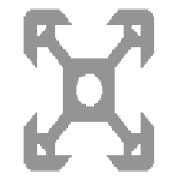
# Autodesk Inventor part: V-slot 20 mm x 20 mm
Saved by Autodesk Inventor 2019 (Build 230136000, 136)
## iProperties
Created: 2018-12-31
Part Number: V-slot 20 mm x 20 mm
Material: Aluminum 6061
Description: V Slot Extrusion
Document SubType Name: Modeling
Designer: Ax
Manufacturer: Openbuilds
Standards Organization: ISO
Language: en-US
Size Designation: 470 mm 2020 V-Slot
Categories: <MemberInstance><Categories><Category DisplayName="Structural Shapes" InternalName="089c4875-fa83-4c05-b084-43b9cc11f5ed" Mnemonic="GRDR"><CategoryParameter DisplayName="Mass per Length Unit" InternalName="0bb95a10-148f-4027-a459-38d7b056702a" Mnemonic="shpmass"/><CategoryParameter DisplayName="Section Area" InternalName="1ff91680-64b0-4202-b9a3-7fd3f94bba3b" Mnemonic="secarea"/><CategoryParameter DisplayName="Radius of Gyration (x)" InternalName="25778675-03e9-40c1-b6a8-4a9ed693320d" Mnemonic="gyrradx"/><CategoryParameter DisplayName="Torsional Rigidity Modulus" InternalName="26c1ec35-5026-4c63-ad0a-751cf684a536" Mnemonic="torrigmod"/><CategoryParameter DisplayName="Distance of the Center of Gravity X-X" InternalName="26c9bdb8-9c79-4b4f-a92e-8e197583c9c4" Mnemonic="grcendistX"/><CategoryParameter DisplayName="Legacy Member ID" InternalName="340afe4f-75d7-48d3-ab7d-943f3c3da468" Mnemonic="LegacyMemberID"/><CategoryParameter DisplayName="Base Length" InternalName="42e34263-8f20-4d0e-ad48-bf1385b87c24" Mnemonic="shplen"/><CategoryParameter DisplayName="Moment of Inertia (y)" InternalName="4b9f58ea-bced-460e-81ea-3d29ca5a49e3" Mnemonic="inermomy"/><CategoryParameter DisplayName="Moment of Inertia (x)" InternalName="4cd780bc-73d7-43ac-917a-579e5cbd684d" Mnemonic="inermomx"/><CategoryParameter DisplayName="Custom Base Point" InternalName="4f1d1b73-316d-484b-a3df-9cbabb16eb77" Mnemonic="shpBasePoint"/><CategoryParameter DisplayName="Shape Height" InternalName="50274e7d-5ac0-4796-92cb-c59e54983c67" Mnemonic="shpheig"/><CategoryParameter DisplayName="Section Module (y)" InternalName="59eaa5e9-d227-48dc-b6c1-6920f96e0f95" Mnemonic="secmody"/><CategoryParameter DisplayName="Section Designation" InternalName="5a64d034-428d-49c8-ba32-7619764de20f" Mnemonic="shpdes"/><CategoryParameter DisplayName="Section Module (x)" InternalName="72cfad18-cf51-4ed4-aaa7-c6b224f8419f" Mnemonic="secmodx"/><CategoryParameter DisplayName="Torsional Section Modulus" InternalName="7c55a8dc-8844-49f9-a867-cc677b30ec9a" Mnemonic="torsecmod"/><CategoryParameter DisplayName="Shape Width" InternalName="7c717d54-a18f-4666-b4d4-573cce22c62c" Mnemonic="shpwdth"/><CategoryParameter DisplayName="Second Shape Thickness" InternalName="9251a8e1-85fd-4e47-af99-afdb762317d9" Mnemonic="shpthick2"/><CategoryParameter DisplayName="FG Authored" InternalName="9c666724-f362-4ea7-ac62-f6a007de5c69" Mnemonic="shpFGAuto"/><CategoryParameter DisplayName="Distance of the Center of Gravity Y-Y" InternalName="bcc4fb17-7af4-436a-8f8c-d0aa3b0248c5" Mnemonic="grcendistY"/><CategoryParameter DisplayName="Radius of Gyration (y)" InternalName="bfa18ebe-1636-4dbe-8d42-b263e0b73184" Mnemonic="gyrrady"/><CategoryParameter DisplayName="Shape Thickness" InternalName="d109cf76-8eb4-42fc-9800-4409734adc67" Mnemonic="shpthick"/><CategoryParameter DisplayName="Coefficient of Shear Displacement" InternalName="de4c90c6-aaa8-468f-a335-6737b311b5d3" Mnemonic="shdispc"/><Category DisplayName="Square/Rectangular Tubes" InternalName="afc8e2d8-05d6-4609-8807-f98a9b7d2ed0" Mnemonic="SQRSHP"><CategoryParameter DisplayName="Section Area" InternalName="2f7f79dd-983c-4263-802a-5b6a1495fdc5" Mnemonic="secarea"/><CategoryParameter DisplayName="Section Module (x)" InternalName="50d965a6-04bf-46b9-8ace-861858d348e6" Mnemonic="secmodx"/><CategoryParameter DisplayName="Section Module (y)" InternalName="5106aeac-54a2-4159-a9af-8933dd39dba2" Mnemonic="secmody"/><CategoryParameter DisplayName="Shape Thickness" InternalName="52712fc5-f4ee-4eda-b3f2-6fce82c26419" Mnemonic="shpthick"/><CategoryParameter DisplayName="Moment of Inertia (y)" InternalName="55ec8510-8276-4c45-8f10-594e0fee7eb3" Mnemonic="inermomy"/><CategoryParameter DisplayName="Radius of Gyration (x)" InternalName="56c89926-a299-4389-a862-ac94c9691272" Mnemonic="gyrradx"/><CategoryParameter DisplayName="Radius" InternalName="5d8d062c-e28e-41c1-98da-8e5fee36da1a" Mnemonic="shprad"/><CategoryParameter DisplayName="Moment of Inertia (x)" InternalName="8c4637b6-6b69-4878-9d5d-26a32185d655" Mnemonic="inermomx"/><CategoryParameter DisplayName="Shape Width" InternalName="8c8a1782-5e80-4d77-858b-304b1c0ad1fd" Mnemonic="shpwdth"/><CategoryParameter DisplayName="Radius of Gyration (y)" InternalName="fa48a7f5-f030-40f9-a60b-de8a845b7104" Mnemonic="gyrrady"/></Category></Category><Category DisplayName="DataType" InternalName="23b78d0f-2648-40c6-8793-ca6db495c9e8" Mnemonic="DATATYPE"><CategoryParameter DisplayName="DisplayName" InternalName="05415f3d-3907-474b-a020-eb9d644f4cf3" Mnemonic="DISPLAYNAME"/><CategoryParameter DisplayName="Standard" InternalName="0c0a119c-1e12-4c84-803f-101930972f5e" Mnemonic="STANDARD"/><CategoryParameter DisplayName="Description" InternalName="13903e3d-64b1-4950-80da-f627842ea37f" Mnemonic="DESCRIPTION"/><CategoryParameter DisplayName="Designation" InternalName="2675968c-4ce5-49e0-a4f5-552d29089031" Mnemonic="DESIGNATION"/><CategoryParameter DisplayName="Default Row" InternalName="2af9ec52-faaa-4026-b378-f9fa4afca842" Mnemonic="DEFAULTROW"/><CategoryParameter DisplayName="Folder Name" InternalName="3f06958e-8713-4116-9be7-ed6184ecc97b" Mnemonic="FOLDERNAME"/><CategoryParameter DisplayName="Revision Guid" InternalName="45a75005-10b1-4dfc-8d6d-dfe629f0b93c" Mnemonic="REVISIONGUID"/><CategoryParameter DisplayName="FileName" InternalName="8b46a4cc-9585-4fed-90c3-899f57e09a73" Mnemonic="FILENAME"/><CategoryParameter DisplayName="StdsOrg" InternalName="8f5914e1-4693-403f-8ab5-d37768198c9d" Mnemonic="STDSORG"/><CategoryParameter DisplayName="Family Version" InternalName="914462f6-6e19-4b14-ba84-155b9680b1d0" Mnemonic="FAMILYREVISION"/><CategoryParameter DisplayName="Standard Revision" InternalName="91d5a463-65c2-4fde-b823-3b7fea5e8e17" Mnemonic="STANDARDREVISION"/><CategoryParameter DisplayName="Member Revision" InternalName="a65d44b9-392f-4f4f-857b-e4b3d54996fe" Mnemonic="MEMBERREVISION"/><CategoryParameter DisplayName="ClipFormat" InternalName="bc51e27b-3422-4e78-93ef-cec197ddf230" Mnemonic="CLIPFORMAT"/><CategoryParameter DisplayName="Manufacturer" InternalName="cd6c7a72-a28a-4e50-99a9-2c7f4e13e5ad" Mnemonic="MANUFACTURER"/><CategoryParameter DisplayName="InternalName" InternalName="cf1d0246-76d9-4b4a-8305-fa0409afb5c1" Mnemonic="INTERNALNAME"/><CategoryParameter DisplayName="IsMetric" InternalName="e2385c5b-1ea4-4823-96a8-8de651266ec3" Mnemonic="ISMETRIC"/><Category DisplayName="Part" InternalName="c0e0b642-3bcb-4cc8-9e80-f96d35c4afa4" Mnemonic="PART"><CategoryParameter DisplayName="Part Number" InternalName="016b6077-bfbe-49bd-92c9-d8d59c39c941" Mnemonic="PARTNUMBER"/><CategoryParameter DisplayName="Stock Number" InternalName="4dba7c1c-e26c-444e-836c-b08b433409a8" Mnemonic="STOCKNUMBER"/><CategoryParameter DisplayName="Material Key" InternalName="5c9a8adb-dd2b-4535-b97f-0a94a95fe41f" Mnemonic="MATERIALKEY"/><CategoryParameter DisplayName="Material" InternalName="818a152a-d3c3-49ca-80ee-df7d91421b8e" Mnemonic="MATERIAL"/></Category></Category></Categories><FamilyTemplate Id="vslot 20 x 20 v2"><FamilyTemplateParameters><FamilyTemplateParameter ObjectType="kModelParameterObject" ValueType="xs:double" Id="12" ObjectReferenceKey="Length"/><FamilyTemplateParameter ObjectType="kModelParameterObject" ValueType="xs:double" Id="13" ObjectReferenceKey="Height"/><FamilyTemplateParameter ObjectType="kModelParameterObject" ValueType="xs:double" Id="14" ObjectReferenceKey="Width"/><FamilyTemplateParameter ObjectType="kPartComponentDefinitionObject" ValueType="xs:string" Id="25" SubObjectId="Material"/><FamilyTemplateParameter ObjectType="kPropertyObject" ValueType="xs:string" Id="28" ObjectReferenceKey="{32853F0F-3444-11d1-9E93-0060B03C1CA6}" SubObjectId="5"/><FamilyTemplateParameter ObjectType="kPropertyObject" ValueType="xs:string" Id="29" ObjectReferenceKey="{32853F0F-3444-11d1-9E93-0060B03C1CA6}" SubObjectId="52"/></FamilyTemplateParameters></FamilyTemplate><CategoryParameterMap><ParamToTemplateMap><ParamToTemplate CategoryParameter="//CategoryParameter[@InternalName='cf1d0246-76d9-4b4a-8305-fa0409afb5c1']" ConstantValue="da8cd6af-c18d-48c7-acef-327f15a6aa53"/><ParamToTemplate CategoryParameter="//CategoryParameter[@InternalName='45a75005-10b1-4dfc-8d6d-dfe629f0b93c']" ConstantValue="3429af54-2f82-4f9b-a0be-007b11a13b69"/><ParamToTemplate CategoryParameter="//CategoryParameter[@InternalName='3f06958e-8713-4116-9be7-ed6184ecc97b']" ConstantValue="vslot 20 x 20 v2"/><ParamToTemplate CategoryParameter="//CategoryParameter[@InternalName='8f5914e1-4693-403f-8ab5-d37768198c9d']" ConstantValue="ISO"/><ParamToTemplate CategoryParameter="//CategoryParameter[@InternalName='0c0a119c-1e12-4c84-803f-101930972f5e']" TemplateParameter="20"/><ParamToTemplate CategoryParameter="//CategoryParameter[@InternalName='91d5a463-65c2-4fde-b823-3b7fea5e8e17']" TemplateParameter="21"/><ParamToTemplate CategoryParameter="//CategoryParameter[@InternalName='cd6c7a72-a28a-4e50-99a9-2c7f4e13e5ad']" ConstantValue="Openbuilds"/><ParamToTemplate CategoryParameter="//CategoryParameter[@InternalName='13903e3d-64b1-4950-80da-f627842ea37f']" ConstantValue="V Slot Extrusion"/><ParamToTemplate CategoryParameter="//CategoryParameter[@InternalName='05415f3d-3907-474b-a020-eb9d644f4cf3']" ConstantValue="vslot 20 x 20 v2"/><ParamToTemplate CategoryParameter="//CategoryParameter[@InternalName='914462f6-6e19-4b14-ba84-155b9680b1d0']" ConstantValue="11"/><ParamToTemplate CategoryParameter="//CategoryParameter[@InternalName='bc51e27b-3422-4e78-93ef-cec197ddf230']" ConstantValue="CF_INVENTOR.STDPARTS"/><ParamToTemplate CategoryParameter="//CategoryParameter[@InternalName='e2385c5b-1ea4-4823-96a8-8de651266ec3']" ConstantValue="true"/><ParamToTemplate CategoryParameter="//CategoryParameter[@InternalName='2af9ec52-faaa-4026-b378-f9fa4afca842']" ConstantValue="1"/><ParamToTemplate CategoryParameter="//CategoryParameter[@InternalName='9c666724-f362-4ea7-ac62-f6a007de5c69']" ConstantValue="1"/><ParamToTemplate CategoryParameter="//CategoryParameter[@InternalName='8b46a4cc-9585-4fed-90c3-899f57e09a73']" ConstantValue="470 mm 2020 V-Slot"/><ParamToTemplate CategoryParameter="//CategoryParameter[@InternalName='a65d44b9-392f-4f4f-857b-e4b3d54996fe']" ConstantValue="44ae6ecb-86cc-4f6a-907d-18f6927daee7"/><ParamToTemplate CategoryParameter="//CategoryParameter[@InternalName='a65d44b9-392f-4f4f-857b-e4b3d54996fe']" ConstantValue="44ae6ecb-86cc-4f6a-907d-18f6927daee7"/><ParamToTemplate CategoryParameter="//CategoryParameter[@InternalName='2675968c-4ce5-49e0-a4f5-552d29089031']" TemplateParameter="29"/><ParamToTemplate CategoryParameter="//CategoryParameter[@InternalName='50274e7d-5ac0-4796-92cb-c59e54983c67']" TemplateParameter="13"/><ParamToTemplate CategoryParameter="//CategoryParameter[@InternalName='42e34263-8f20-4d0e-ad48-bf1385b87c24']" TemplateParameter="12"/><ParamToTemplate CategoryParameter="//CategoryParameter[@InternalName='818a152a-d3c3-49ca-80ee-df7d91421b8e']" TemplateParameter="25"/><ParamToTemplate CategoryParameter="//CategoryParameter[@InternalName='016b6077-bfbe-49bd-92c9-d8d59c39c941']" TemplateParameter="28"/><ParamToTemplate CategoryParameter="//CategoryParameter[@InternalName='7c717d54-a18f-4666-b4d4-573cce22c62c']" TemplateParameter="14"/></ParamToTemplateMap></CategoryParameterMap></MemberInstance>
Mass: 8.74677 g
Surface Area: 40.0875 cm^2
Volume: 3.22759 cm^3
Density: 2.71 g/cm^3
Appearance: Aluminum - Flat
IsCustomPart: 0
Author: Ax
G_L: 470.000 mm
Autodesk Inventor part; units mm, degrees
ref_plane "YZ Plane" through (0, 0, 0) normal (1, 0, 0) x (0, 1, 0)
ref_plane "XZ Plane" through (0, 0, 0) normal (0, 1, 0) x (-1, 0, 0)
ref_plane "Start Plane" through (0, 0, 0) normal (0, 0, 1) x (1, 0, 0)
ref_plane "End Plane" through (0, 0, 470) normal (0, 0, 1) x (1, 0, 0)
sketch "Sketch1" plane through (0, 0, 0) normal (0, 0, 1) x (1, 0, 0)
  line L0 (10, -4.5951) -> (10, -8.2)
  line L1 (-10, -8.2) -> (-10, -4.5951)
  line L2 (-10, 10) -> (10, -10) construction
  line L3 (10, 10) -> (-10, -10) construction
  circle A0 centre (0, 0) radius 2.1
  line L4 (-2.84, -3.9007) -> (2.84, -3.9007)
  line L5 (3.9007, -2.84) -> (3.9007, 2.84)
  line L6 (2.84, 3.9007) -> (-2.84, 3.9007)
  line L7 (-3.9007, 2.84) -> (-3.9007, -2.84)
  line L8 (-3.9007, -3.9007) -> (3.9007, 3.9007) construction
  line L9 (3.9007, -3.9007) -> (-3.9007, 3.9007) construction
  line L10 (-3.9007, -2.84) -> (-2.84, -3.9007) construction
  line L11 (-2.84, -3.9007) -> (-5.4993, -6.56)
  line L12 (-5.4993, -6.56) -> (-5.4993, -8.2)
  line L13 (-5.4993, -8.2) -> (-2.7951, -8.2)
  line L14 (-2.7951, -8.2) -> (-4.5951, -10)
  line L15 (0, 0) -> (0, -3.9007) construction
  line L16 (3.9007, -2.84) -> (2.84, -3.9007) construction
  line L17 (2.84, -3.9007) -> (5.4993, -6.56)
  line L18 (5.4993, -6.56) -> (5.4993, -8.2)
  line L19 (5.4993, -8.2) -> (2.7951, -8.2)
  line L20 (2.7951, -8.2) -> (4.5951, -10)
  line L21 (-2.84, -3.9007) -> (-3.9007, -2.84) construction
  line L22 (-3.9007, -2.84) -> (-6.56, -5.4993)
  line L23 (-6.56, -5.4993) -> (-8.2, -5.4993)
  line L24 (-8.2, -5.4993) -> (-8.2, -2.7951)
  line L25 (-8.2, -2.7951) -> (-10, -4.5951)
  line L26 (3.9007, -2.84) -> (6.56, -5.4993)
  line L27 (6.56, -5.4993) -> (8.2, -5.4993)
  line L28 (8.2, -5.4993) -> (8.2, -2.7951)
  line L29 (8.2, -2.7951) -> (10, -4.5951)
  arc A1 (-10, -8.2) -> (-8.2, -10) centre (-8.2, -8.2) ccw
  arc A2 (8.2, -10) -> (10, -8.2) centre (8.2, -8.2) ccw
  line L30 (-8.2, -6.56) -> (-7.7111, -6.56)
  line L31 (-6.6505, -8.2) -> (-8.2, -8.2)
  line L32 (-8.2, -8.2) -> (-8.2, -6.56)
  line L33 (-6.6505, -7.6207) -> (-7.7111, -6.56)
  line L34 (-6.6505, -7.6207) -> (-6.6505, -8.2)
  line L35 (8.2, -6.56) -> (7.7111, -6.56)
  line L36 (6.6505, -8.2) -> (8.2, -8.2)
  line L37 (8.2, -8.2) -> (8.2, -6.56)
  line L38 (6.6505, -7.6207) -> (7.7111, -6.56)
  line L39 (6.6505, -7.6207) -> (6.6505, -8.2)
  line L40 (8.2, -10) -> (4.5951, -10)
  line L41 (-4.5951, -10) -> (-8.2, -10)
  line L42 (-3.9007, 0) -> (3.9007, 0) construction
  line L43 (10, 4.5951) -> (10, 8.2)
  line L44 (-10, 8.2) -> (-10, 4.5951)
  line L45 (-2.84, 3.9007) -> (2.84, 3.9007)
  line L46 (-3.9007, 2.84) -> (-2.84, 3.9007) construction
  line L47 (-2.84, 3.9007) -> (-5.4993, 6.56)
  line L48 (-5.4993, 6.56) -> (-5.4993, 8.2)
  line L49 (-5.4993, 8.2) -> (-2.7951, 8.2)
  line L50 (-2.7951, 8.2) -> (-4.5951, 10)
  line L51 (2.84, 3.9007) -> (5.4993, 6.56)
  line L52 (5.4993, 6.56) -> (5.4993, 8.2)
  line L53 (5.4993, 8.2) -> (2.7951, 8.2)
  line L54 (2.7951, 8.2) -> (4.5951, 10)
  line L55 (3.9007, 2.84) -> (2.84, 3.9007) construction
  line L56 (-8.2, 2.7951) -> (-10, 4.5951)
  line L57 (-2.84, 3.9007) -> (-3.9007, 2.84) construction
  line L58 (-3.9007, 2.84) -> (-6.56, 5.4993)
  line L59 (-6.56, 5.4993) -> (-8.2, 5.4993)
  line L60 (-8.2, 5.4993) -> (-8.2, 2.7951)
  line L61 (3.9007, 2.84) -> (6.56, 5.4993)
  line L62 (6.56, 5.4993) -> (8.2, 5.4993)
  line L63 (8.2, 5.4993) -> (8.2, 2.7951)
  line L64 (8.2, 2.7951) -> (10, 4.5951)
  arc A3 (-8.2, 10) -> (-10, 8.2) centre (-8.2, 8.2) ccw
  arc A4 (10, 8.2) -> (8.2, 10) centre (8.2, 8.2) ccw
  line L65 (-8.2, 6.56) -> (-7.7111, 6.56)
  line L66 (-6.6505, 8.2) -> (-8.2, 8.2)
  line L67 (-8.2, 8.2) -> (-8.2, 6.56)
  line L68 (-6.6505, 7.6207) -> (-7.7111, 6.56)
  line L69 (-6.6505, 7.6207) -> (-6.6505, 8.2)
  line L70 (8.2, 6.56) -> (7.7111, 6.56)
  line L71 (6.6505, 7.6207) -> (7.7111, 6.56)
  line L72 (8.2, 8.2) -> (8.2, 6.56)
  line L73 (6.6505, 7.6207) -> (6.6505, 8.2)
  line L74 (6.6505, 8.2) -> (8.2, 8.2)
  line L75 (8.2, 10) -> (4.5951, 10)
  line L76 (-4.5951, 10) -> (-8.2, 10)
  line L77 (-8.2, 10) -> (-4.5951, 10)
  line L78 (4.5951, 10) -> (8.2, 10)
  point P0 (8.2, -8.2)
  point P1 (0, 3.9007)
  point P2 (8.2, 8.2)
  dimension "Width" = 20
  dimension "Height" = 20
  dimension "d2" = 4.2
  dimension "d3" = 1.5
  dimension "d4" = 1.64
  dimension "d6" = 5.68
  dimension "d7" = 1.8
  dimension "d9" = 1.5
  constraints: 158 end point, 60 symmetric about line, 12 parallel, 8 midpoint, 8 point on circle, 6 perpendicular, 6 tangent, 5 centre point, 5 horizontal, 5 point on line, 1 coincident, 1 equal radius, 2 other
  measures "Width" distance of L2.end L3.end
  measures "Height" distance of L3.start L2.end
  measures "d2" diameter of A0
  measures "d3" distance of L4.start L7.end
  measures "d4" distance of L11.end L12.end
  measures "d6" distance of L4.start L4.end
  measures "d7" radius of A1
  measures "d9" distance of L30.end L33.start
extrude "Body" add sketch "Sketch1" along normal up to surface (470 mm away) from surface at 0
sketch "Sketch4" plane through (0, 0, 0) normal (0, 0, 1) x (1, 0, 0)
  line L0 (0, 0) -> (10, 0)
ref_plane "Work Plane4" through (0, 0, 0) normal (0, -1, 0) x (1, 0, 0)
sketch "Sketch5" plane through (0, 0, 0) normal (0, -1, 0) x (1, 0, 0)
  line L0 (-2, 0) -> (12, 0) construction
  line L1 (-2, 470) -> (12, 470) construction
  dimension "d17" = 470
  measures "d17" distance between parallel lines of L0 L1
equation "\"G_OFFSET_START\" = 0"
equation "\"G_OFFSET_END\" = 0"
equation "\"G_L\" = d17"
body "Solid1"
